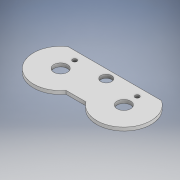
# Autodesk Inventor part: paitent remote top
Saved by Autodesk Inventor 2021 (Build 250183000, 183)
## iProperties
Created: 2023-01-12
Part Number: paitent remote top
Material: Generic
Document SubType Name: Modeling
Designer: boyle
Density: 1 g/cm^3
Appearance: Default
Author: boyle
Autodesk Inventor part; units mm, degrees
ref_plane "YZ Plane" through (0, 0, 0) normal (1, 0, 0) x (0, 1, 0)
ref_plane "XZ Plane" through (0, 0, 0) normal (0, 1, 0) x (-1, 0, 0)
ref_plane "XY Plane" through (0, 0, 0) normal (0, 0, 1) x (1, 0, 0)
sketch "Sketch1" plane through (0, 0, 0) normal (0, 1, 0) x (-1, 0, 0)
  line L0 (-23.3466, 0) -> (-154.4106, 0)
  line L1 (-102.87, 54.61) -> (-74.9238, 54.61)
  line L2 (-88.9, 0) -> (-23.3466, 0)
  line L3 (-88.9, 0) -> (-154.4106, 0)
  arc A0 (-102.87, 54.61) -> (-154.4106, 0) centre (-133.35, 31.75) ccw
  arc A1 (-23.3466, 0) -> (-74.9238, 54.61) centre (-44.4805, 31.7012) ccw
  point P0 (0, 0)
  dimension "d0" = 76.2
  dimension "d1" = 76.2
  dimension "d2" = 131.064
  dimension "d12" = 54.61
  constraints: 8 end point, 4 point on circle, 2 centre point, 2 collinear, 1 horizontal, 1 parallel, 1 point on line
  measures "d0" diameter of A0
  measures "d1" diameter of A1
  measures "d2" distance of L0.start L0.end
  measures "d12" distance from line of L1 L2.start
extrude "Extrusion1" add sketch "Sketch1" along normal blind 4.826
sketch "Sketch2" plane through (0, 4.826, 0) normal (0, 1, 0) x (1, 0, 0)
  line L0 (154.4106, 0) -> (23.3466, 0) projected
  arc A0 (23.3466, 0) -> (74.9238, -54.61) centre (44.4805, -31.7012) ccw projected
  line L1 (74.9238, -54.61) -> (102.87, -54.61) projected
  arc A1 (102.87, -54.61) -> (154.4106, 0) centre (133.35, -31.75) ccw projected
  circle A2 centre (44.4805, -31.7012) radius 9.525
  circle A3 centre (133.35, -31.75) radius 9.525
  line L2 (88.8786, 0) -> (88.8969, -54.61)
  line L3 (88.891, -24.1125) -> (88.8786, 0)
  circle A4 centre (132.3699, -12.0338) radius 3
  circle A5 centre (44.4805, -12.0338) radius 3
  circle A6 centre (88.8848, -12.0563) radius 7.5
  point P0 (0, 0)
  dimension "d9" = 6
  dimension "d10" = 6
  dimension "d11" = 15
  constraints: 5 centre point, 4 end point, 3 midpoint, 2 coincident
  measures "d9" diameter of A4
  measures "d10" diameter of A5
  measures "d11" diameter of A6
extrude "Extrusion2" cut sketch "Sketch2" against normal through all contours A6 L2 | L2 A6 | A2 | A3 | A4 | A5
body "Solid1"
